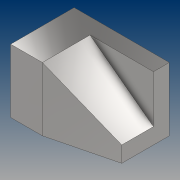
# Autodesk Inventor part: 50
Saved by Autodesk Inventor 2020.2 (Build 242310000, 310)
## iProperties
Created: 2020-09-17
Part Number: 50
Material: 鋼、碳鋼
Document SubType Name: Modeling
Designer: user
Density: 7.85 g/cm^3
Appearance: 半拋光
Mass: 580.9 g
Surface Area: 116.808 cm^2
Volume: 74 cm^3
Author: user
Autodesk Inventor part; units mm, degrees
ref_plane "YZ Plane" through (0, 0, 0) normal (1, 0, 0) x (0, 1, 0)
ref_plane "XZ Plane" through (0, 0, 0) normal (0, 1, 0) x (-1, 0, 0)
sketch "草圖1" plane through (0, 0, 0) normal (0, 1, 0) x (-1, 0, 0)
  line L0 (0, 0) -> (-60, 0)
  line L1 (-60, 0) -> (-60, 40)
  line L2 (-60, 40) -> (0, 40)
  line L3 (0, 40) -> (0, 0)
  dimension "d0" = 60
  dimension "d1" = 40
  constraints: 8 end point, 2 parallel, 1 horizontal, 1 perpendicular
  measures "d0" distance of L1.end L2.end
  measures "d1" distance of L2.end L0.start
extrude "擠出1" add sketch "草圖1" along normal blind 40
sketch "草圖2" plane through (0, 40, 0) normal (0, 1, 0) x (1, 0, 0)
  line L0 (60, -40) -> (0, -40) projected
  line L1 (0, -40) -> (0, 0) projected
  line L2 (0, 0) -> (60, 0) projected
  line L3 (60, 0) -> (60, -40) projected
  line L4 (0, -40) -> (60, -40) projected
  line L5 (20, -40) -> (60, -30)
  dimension "d4" = 30
  dimension "d5" = 20
  constraints: 2 end point, 2 point on line
  measures "d4" distance from line of L2 L5.end
  measures "d5" distance from line of L5.start L1
extrude "擠出2" cut sketch "草圖2" against normal through all contours L0 L5 L3
sketch "草圖3" plane through (60, 0, 0) normal (1, 0, 0) x (0, 0, -1)
  line L0 (0, 40) -> (0, 0) construction
  line L1 (0, 0) -> (-30, 0) construction
  line L2 (-30, 0) -> (-30, 40) construction
  line L3 (-30, 40) -> (0, 40) construction
  line L4 (-40, 0) -> (-40, 40) construction
  line L5 (-40, 40) -> (-30, 10)
  line L6 (-30, 10) -> (-10, 10)
  line L7 (-30, 40) -> (-30, 0) construction
  line L8 (-10, 10) -> (-10, 40)
  line L9 (0, 40) -> (-40, 40) construction
  line L10 (-10, 40) -> (-40, 40)
  dimension "d8" = 10
  dimension "d9" = 10
  dimension "d10" = 30
  constraints: 8 end point, 2 perpendicular, 1 collinear, 1 point on line
  measures "d8" distance between parallel lines of L1 L6
  measures "d9" distance between parallel lines of L8 L0
  measures "d10" distance from line of L0 L5.end
ref_plane "工作平面1" through (20, 40, 40) normal (-1, 0, 0) x (0, 0, 1)
sketch "草圖4" plane through (20, 40, 40) normal (-1, 0, 0) x (0, 0, 1)
  line L0 (-40, -40) -> (-40, 0) construction
  line L1 (-40, 0) -> (0, 0) construction
  line L2 (0, 0) -> (0, -40) construction
  line L3 (0, -40) -> (-40, -40) construction
  line L4 (0, 19.9145) -> (-30, 19.9145)
  line L5 (-30, 19.9145) -> (-30, 0)
  line L6 (-30, 0) -> (0, 0)
  line L7 (0, 0) -> (0, 19.9145)
  line L8 (0, -40) -> (0, 0) projected
  dimension "d11" = 10
  constraints: 8 end point, 2 collinear, 2 parallel, 1 horizontal, 1 perpendicular
  measures "d11" distance between parallel lines of L0 L5
loft "斷面混成1" cut profiles "草圖3", "草圖4"
